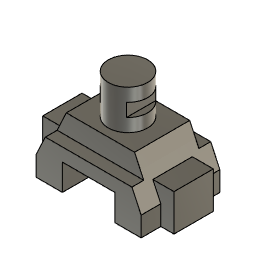
Sketch10_Final v0 (Autodesk Fusion 360 design; units mm, degrees)
Autodesk Fusion 360 part; units mm, degrees
sketch "Sketch1" plane through (0, 0, 0) normal (0, 1, 0) x (1, 0, 0)
  line L0 (20, 0) -> (40, 0)
  line L1 (40, 0) -> (40, -15)
  line L2 (26, -45) -> (0, -45)
  line L3 (-26, -45) -> (0, -45)
  line L4 (-40, 0) -> (-40, -15)
  line L5 (-20, 0) -> (-40, 0)
  line L6 (20, -20) -> (-20, -20)
  line L7 (-20, -20) -> (-20, 0)
  line L8 (20, 0) -> (20, -20)
  line L9 (-40, 0) -> (-40, -15)
  line L10 (0, -45) -> (-26, -45)
  line L11 (-40, -15) -> (-26, -45)
  line L12 (40, -15) -> (26, -45)
  dimension "d5" = 15
  dimension "d6" = 26
  constraint horizontal L0
  constraint vertical L1
  constraint horizontal L2
  constraint horizontal L6
  constraint perpendicular L6 L7
  constraint parallel L7 L8
  constraint perpendicular L5 L9
  measures "d5" distance of L4.start L4.end
  measures "d6" distance of L2.end L3.start
extrude "Extrude1" add sketch "Sketch1" along normal mid plane 60
sketch "Sketch3" plane through (0, 0, 0) normal (1, 0, 0) x (0, 1, 0)
  line L0 (-30, 45) -> (-21, 45)
  line L1 (-21, 45) -> (-21, 30)
  line L2 (-21, 30) -> (-30, 30)
  line L3 (-30, 30) -> (-30, 45)
  line L4 (21, 45) -> (21, 30)
  line L5 (21, 30) -> (30, 30)
  line L6 (30, 30) -> (30, 45)
  line L7 (30, 45) -> (21, 45)
  dimension "d9" = 9
  dimension "d10" = 15
  constraint horizontal L0
  constraint vertical L1
  constraint horizontal L2
  constraint vertical L3
  measures "d9" distance of L0.start L0.end
  measures "d10" distance of L0.start L2.end
extrude "Extrude2" cut sketch "Sketch3" along normal mid plane 120
sketch "Sketch4" plane through (0, 0, 45) normal (0, 0, 1) x (-1, 0, 0)
  line L0 (-26, -21) -> (26, -21)
  line L1 (26, -21) -> (26, 21)
  line L2 (26, 21) -> (-26, 21)
  line L3 (-26, 21) -> (-26, -21)
  line L4 (40, 30) -> (40, 15)
  line L5 (40, 15) -> (50, 15)
  line L6 (50, 15) -> (50, -15)
  line L7 (50, -15) -> (40, -15)
  line L8 (40, -15) -> (28, -15)
  line L9 (28, -15) -> (28, 15)
  line L10 (28, 15) -> (40, 15)
  line L11 (-50, 15) -> (-50, -15)
  line L12 (-50, -15) -> (-40, -15)
  line L13 (-40, -15) -> (-28, -15)
  line L14 (-28, -15) -> (-28, 15)
  line L15 (-28, 15) -> (-40, 15)
  line L16 (-40, 15) -> (-50, 15)
  dimension "d13" = 15
  dimension "d14" = 10
  dimension "d15" = 30
  constraint vertical L4
  constraint horizontal L5
  constraint vertical L6
  constraint horizontal L7
  constraint horizontal L8
  constraint vertical L9
  constraint horizontal L10
  measures "d13" distance of L4.start L4.end
  measures "d14" distance of L4.end L5.end
  measures "d15" distance of L4.end L7.end
extrude "Extrude3" add sketch "Sketch4" along normal blind 28 from surface at -45 contours L5 L6 L7 L8 L9 L10 | L11 L12 L13 L14 L15 L16
sketch "Sketch5" plane through (0, 0, 45) normal (0, 0, 1) x (-1, 0, 0)
  line L0 (-26, -21) -> (26, -21)
  line L1 (26, -21) -> (26, 21)
  line L2 (26, 21) -> (-26, 21)
  line L3 (-26, 21) -> (-26, -21)
  circle A0 centre (0, 0) radius 15
  dimension "d19" = 30
  constraint coincident A0.centre origin
  measures "d19" diameter of A0
extrude "Extrude4" add sketch "Sketch5" along normal blind 30 contours A0
sketch "Sketch6" plane through (0, 0, 0) normal (0, 1, 0) x (-1, 0, 0)
  line L0 (-10, 55) -> (-10, 65)
  line L1 (-10, 55) -> (-18, 55)
  line L2 (-18, 55) -> (-18, 65)
  line L3 (-18, 65) -> (-10, 65)
  line L4 (-10, 65) -> (-10, 55)
  line L5 (18, 55) -> (18, 65)
  line L6 (10, 55) -> (18, 55)
  line L7 (10, 65) -> (10, 55)
  line L8 (18, 65) -> (10, 65)
  constraint vertical L0
  constraint horizontal L1
  constraint vertical L2
  constraint horizontal L3
  constraint vertical L4
extrude "Extrude5" cut sketch "Sketch6" along normal mid plane 60
